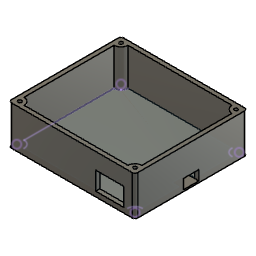
PageTurner_Housing (Autodesk Fusion 360 design; units mm, degrees)
Autodesk Fusion 360 part; units mm, degrees
note: some values were not read from the file. Set by a fixed rule: which sketch regions a step uses.
sketch "Skizze1" plane through (0, 0, 0) normal (0, 1, 0) x (1, 0, 0)
  line L0 (0, 0) -> (90, 0)
  line L1 (90, 0) -> (90, -80)
  line L2 (90, -80) -> (0, -80)
  line L3 (0, -80) -> (0, 0)
  dimension "d1" = 90
  dimension "d2" = 80
  constraint horizontal L0
  constraint vertical L1
  constraint horizontal L2
  constraint vertical L3
  constraint coincident L0.start L3.end
  measures "d1" distance of L0.start L0.end
  measures "d2" distance of L0.start L2.end
sketch "Skizze2" plane through (45, 0, 40) normal (0, 1, 0) x (1, 0, 0)
extrude "Extrusion1" add sketch "Skizze1" along normal blind 28
sketch "Skizze3" plane through (0, 0, 80) normal (0, 0, 1) x (1, 0, 0)
  line L0 (0, 0) -> (90, 0)
  line L1 (90, 0) -> (90, 28)
  line L2 (90, 28) -> (0, 28)
  line L3 (0, 28) -> (0, 0)
  line L4 (62, 16.5) -> (82, 16.5)
  line L5 (82, 16.5) -> (82, 3.5)
  line L6 (82, 3.5) -> (62, 3.5)
  line L7 (62, 3.5) -> (62, 16.5)
  dimension "d6" = 20
  dimension "d7" = 13
  dimension "d8" = 3.5
  dimension "d9" = 8
  constraint horizontal L4
  constraint vertical L5
  constraint horizontal L6
  constraint vertical L7
  measures "d6" distance of L4.start L4.end
  measures "d7" distance of L4.start L6.end
  measures "d8" vertical distance of L0.end L5.end
  measures "d9" horizontal distance of L1.end L4.end
extrude "Extrusion2" cut sketch "Skizze3" against normal blind 8 contours L4 L5 L6 L7
sketch "Skizze4" plane through (90, 0, 0) normal (1, 0, 0) x (0, 0, -1)
  line L0 (-80, 0) -> (0, 0)
  line L1 (0, 0) -> (0, 28)
  line L2 (0, 28) -> (-80, 28)
  line L3 (-80, 28) -> (-80, 0)
  line L4 (-45.5, 8.1) -> (-34.5, 8.1)
  line L5 (-34.5, 8.1) -> (-34.5, 1.1)
  line L6 (-34.5, 1.1) -> (-45.5, 1.1)
  line L7 (-45.5, 1.1) -> (-45.5, 8.1)
  dimension "d12" = 11
  dimension "d13" = 7
  dimension "d14" = 34.5
  dimension "d15" = 1.1
  constraint horizontal L4
  constraint vertical L5
  constraint horizontal L6
  constraint vertical L7
  measures "d12" distance of L4.start L4.end
  measures "d13" distance of L4.start L6.end
  measures "d14" horizontal distance of L0.start L6.end
  measures "d15" vertical distance of L0.start L6.end
extrude "Extrusion3" cut sketch "Skizze4" against normal blind 8 contours L4 L5 L6 L7
sketch "Skizze5" plane through (0, 28, 0) normal (0, 1, 0) x (-1, 0, 0)
  line L0 (0, 80) -> (-90, 80)
  line L1 (-90, 80) -> (-90, 0)
  line L2 (-90, 0) -> (0, 0)
  line L3 (0, 0) -> (0, 80)
  circle A0 centre (-4, 4) radius 1.25
  dimension "d26" = 2.5
  dimension "d27" = 4
  dimension "d28" = 4
  measures "d26" diameter of A0
  measures "d27" horizontal distance of L2.end A0.centre
  measures "d28" vertical distance of L2.end A0.centre
extrude "Extrusion4" cut sketch "Skizze5" against normal blind 20 contours A0
sketch "Skizze6" plane through (0, 28, 0) normal (0, 1, 0) x (-1, 0, 0)
  circle A0 centre (-4, 4) radius 1.25
  line L0 (0, 80) -> (-90, 80)
  line L1 (-90, 80) -> (-90, 0)
  line L2 (-90, 0) -> (0, 0)
  line L3 (0, 0) -> (0, 80)
  circle A1 centre (-86, 4) radius 1.25
  dimension "d31" = 2.5
  dimension "d32" = 4
  dimension "d33" = 4
  measures "d31" diameter of A1
  measures "d32" horizontal distance of L1.end A1.centre
  measures "d33" vertical distance of L1.end A1.centre
extrude "Extrusion5" cut sketch "Skizze6" against normal blind 20 contours A1
sketch "Skizze7" plane through (0, 28, 0) normal (0, 1, 0) x (-1, 0, 0)
  circle A0 centre (-86, 4) radius 1.25
  circle A1 centre (-4, 4) radius 1.25
  line L0 (0, 80) -> (-90, 80)
  line L1 (-90, 80) -> (-90, 0)
  line L2 (-90, 0) -> (0, 0)
  line L3 (0, 0) -> (0, 80)
  circle A2 centre (-86, 76) radius 1.25
  dimension "d36" = 2.5
  dimension "d37" = 4
  dimension "d38" = 4
  measures "d36" diameter of A2
  measures "d37" vertical distance of L0.end A2.centre
  measures "d38" horizontal distance of L0.end A2.centre
extrude "Extrusion6" cut sketch "Skizze7" against normal blind 20 contours A2
sketch "Skizze8" plane through (0, 28, 0) normal (0, 1, 0) x (-1, 0, 0)
  circle A0 centre (-86, 76) radius 1.25
  circle A1 centre (-86, 4) radius 1.25
  circle A2 centre (-4, 4) radius 1.25
  line L0 (0, 80) -> (-90, 80)
  line L1 (-90, 80) -> (-90, 0)
  line L2 (-90, 0) -> (0, 0)
  line L3 (0, 0) -> (0, 80)
  circle A3 centre (-4, 76) radius 1.25
  dimension "d41" = 2.5
  dimension "d42" = 4
  dimension "d43" = 4
  measures "d41" diameter of A3
  measures "d42" horizontal distance of L0.start A3.centre
  measures "d43" vertical distance of L0.start A3.centre
extrude "Extrusion7" cut sketch "Skizze8" against normal blind 20 contours A3
fillet "Abrundung5" radius 2 4 edges at (90, 14, 80) (90, 14, 0) (0, 14, 0) (0, 14, 80)
sketch "Skizze9" plane through (0, 28, 0) normal (0, 1, 0) x (-1, 0, 0)
  arc A0 (0, 78) -> (-2, 80) centre (-2, 78) ccw
  line L0 (-2, 80) -> (-88, 80)
  arc A1 (-88, 80) -> (-90, 78) centre (-88, 78) ccw
  line L1 (-90, 78) -> (-90, 2)
  arc A2 (-90, 2) -> (-88, 0) centre (-88, 2) ccw
  line L2 (-88, 0) -> (-2, 0)
  arc A3 (-2, 0) -> (0, 2) centre (-2, 2) ccw
  line L3 (0, 2) -> (0, 78)
  circle A4 centre (-4, 76) radius 1.25
  circle A5 centre (-86, 76) radius 1.25
  circle A6 centre (-86, 4) radius 1.25
  circle A7 centre (-4, 4) radius 1.25
  line L4 (-8, 77) -> (-82, 77)
  line L5 (-87, 72) -> (-87, 8)
  line L6 (-82, 3) -> (-8, 3)
  line L7 (-3, 8) -> (-3, 72)
  arc A8 (-3, 8) -> (-8, 3) centre (-2.875, 2.875) ccw
  arc A9 (-82, 3) -> (-87, 8) centre (-87.125, 2.875) ccw
  arc A10 (-87, 72) -> (-82, 77) centre (-87.1266, 77.1266) ccw
  arc A11 (-8, 77) -> (-3, 72) centre (-2.8918, 77.1082) ccw
  dimension "d50" = 74
  dimension "d51" = 64
  dimension "d52" = 74
  dimension "d53" = 64
  dimension "d54" = 3
  dimension "d55" = 3
  dimension "d56" = 3
  dimension "d57" = 3
  constraint horizontal L4
  constraint parallel L1 L5
  constraint parallel L2 L6
  constraint parallel L3 L7
  measures "d50" distance of L6.start L6.end
  measures "d51" distance of L7.start L7.end
  measures "d52" distance of L4.start L4.end
  measures "d53" distance of L5.start L5.end
  measures "d54" vertical distance of A0.end L4.start
  measures "d55" horizontal distance of A3.end L7.start
  measures "d56" vertical distance of L2.end L6.end
  measures "d57" horizontal distance of L1.end L5.end
extrude "Extrusion8" cut sketch "Skizze9" against normal blind 26.5 contours L4 L5 L6 L7 A8 A9 A10 A11
sketch "Skizze10" plane through (0, 1.5, 0) normal (0, 1, 0) x (-1, 0, 0)
  line L0 (-87, 45.5) -> (-82, 45.5)
  line L1 (-82, 45.5) -> (-82, 34.5)
  line L2 (-82, 34.5) -> (-87, 34.5)
  line L3 (-87, 34.5) -> (-87, 8)
  line L4 (-82, 3) -> (-8, 3)
  line L5 (-8, 77) -> (-82, 77)
  line L6 (-87, 72) -> (-87, 45.5)
  line L7 (-3, 8) -> (-3, 72)
  arc A0 (-82, 3) -> (-87, 8) centre (-87.125, 2.875) ccw
  arc A1 (-3, 8) -> (-8, 3) centre (-2.875, 2.875) ccw
  arc A2 (-8, 77) -> (-3, 72) centre (-2.8918, 77.1082) ccw
  arc A3 (-87, 72) -> (-82, 77) centre (-87.1266, 77.1266) ccw
